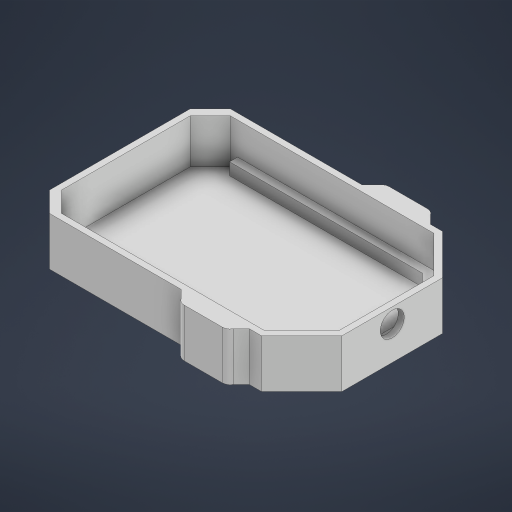
# Autodesk Inventor part: RC5 Controller
Saved by Autodesk Inventor 2024 (Build 280153000, 153)
## iProperties
Created: 2024-03-14
Part Number: RC5 Controller
Material: Generic
Document SubType Name: Modeling
Designer: MenMe
Density: 1 g/cm^3
Appearance: Default
Author: MenMe
Autodesk Inventor part; units mm, degrees
ref_plane "YZ Plane" through (0, 0, 0) normal (1, 0, 0) x (0, 1, 0)
ref_plane "XZ Plane" through (0, 0, 0) normal (0, 1, 0) x (-1, 0, 0)
ref_plane "XY Plane" through (0, 0, 0) normal (0, 0, 1) x (1, 0, 0)
sketch "Sketch1" plane through (0, 0, 0) normal (0, 1, 0) x (-1, 0, 0)
  line L0 (67.75, 0) -> (67.75, -45)
  line L1 (67.75, -45) -> (10, -45)
  line L2 (10, -45) -> (0, -35)
  line L3 (0, -35) -> (0, -10)
  line L4 (0, -10) -> (10, 0)
  line L5 (67.75, 0) -> (10, 0)
  line L6 (28, 0) -> (28, 3)
  line L7 (28, 3) -> (15, 3)
  line L8 (15, 3) -> (15, 0)
  line L9 (28, -45) -> (28, -48)
  line L10 (28, -48) -> (15, -48)
  line L11 (15, -48) -> (15, -45)
  line L12 (58, -48) -> (45, -48)
  line L13 (58, -45) -> (58, -48)
  line L14 (45, -48) -> (45, -45)
  line L15 (58, 0) -> (58, 3)
  line L16 (58, 3) -> (45, 3)
  line L17 (45, 3) -> (45, 0)
  point P0 (0, 0)
  point P1 (21.5, -48)
  point P2 (51.5, -48)
  dimension "d0" = 45
  dimension "d4" = 45
  dimension "d5" = 45
  dimension "d6" = 25
  dimension "d24" = 5
  dimension "d25" = 13
  dimension "d26" = 3
  dimension "d34" = 3
  dimension "d83" = 5
  dimension "d145" = 67.75
  dimension "d148" = 30
  dimension "d155" = 30
  constraints: 36 end point, 8 perpendicular, 6 point on line, 2 equal length, 2 horizontal, 1 midpoint, 16 other
  measures "d0" distance of L0.start L0.end
  measures "d4" angle of L2 L3
  measures "d5" angle of L4 L3
  measures "d6" distance of L2.end L3.end
  measures "d24" distance from line of L1.end L11
  measures "d25" distance of L9.end L10.end
  measures "d26" distance from line of L1 point (21.5, -48)
  measures "d34" distance between parallel lines of L5 L7
  measures "d83" distance from line of L4.end L8
  measures "d145" distance between parallel lines of L0 L3
  measures "d148" distance of L9.end L12.start
  measures "d155" distance of L6.start L15.start
extrude "Extrusion1" add sketch "Sketch1" along normal blind 12 contours L0 L1 L2 L3 L4 L5 | L5 L8 L7 L6 | L9 L10 L11 L1
sketch "Sketch2" plane through (0, 12, 0) normal (0, 1, 0) x (1, 0, 0)
  line L0 (-67.75, 0) -> (-28, 0) projected
  line L1 (-28, 0) -> (-28, -3) projected
  line L2 (-28, -3) -> (-15, -3) projected
  line L3 (-15, -3) -> (-15, 0) projected
  line L4 (-15, 0) -> (-10, 0) projected
  line L5 (-10, 0) -> (0, 10) projected
  line L6 (0, 10) -> (0, 35) projected
  line L7 (0, 35) -> (-10, 45) projected
  line L8 (-10, 45) -> (-15, 45) projected
  line L9 (-15, 45) -> (-15, 48) projected
  line L10 (-15, 48) -> (-28, 48) projected
  line L11 (-28, 48) -> (-28, 45) projected
  line L12 (-28, 45) -> (-67.75, 45) projected
  line L13 (-67.75, 45) -> (-67.75, 0) projected
  line L14 (0, 35) -> (-10, 45) construction
  line L15 (-67.75, 0) -> (-28, 0) construction
  line L16 (-66.25, 43.5) -> (-66.25, 1.5)
  line L17 (-66.25, 1.5) -> (-10.6213, 1.5)
  line L18 (-10.6213, 1.5) -> (-1.5, 10.6213)
  line L19 (-1.5, 10.6213) -> (-1.5, 34.3787)
  line L20 (-1.5, 34.3787) -> (-10.6213, 43.5)
  line L21 (-10.6213, 43.5) -> (-66.25, 43.5)
  line L22 (-10, 0) -> (0, 10) construction
  point P0 (0, 0)
  point P1 (-40, 0)
  point P2 (-66.25, 22.5)
  point P3 (-67.75, 22.5)
  dimension "d126" = 42
  dimension "d132" = 1.5
  dimension "d133" = 1.5
  dimension "d134" = 1.5
  constraints: 12 end point, 4 parallel, 3 perpendicular, 2 midpoint, 1 horizontal alignment, 1 vertical
  measures "d126" distance between parallel lines of L21 L17
  measures "d132" distance between parallel lines of L13 L16
  measures "d133" distance between parallel lines of L6 L19
  measures "d134" distance between parallel lines of L7 L20
extrude "Extrusion2" cut sketch "Sketch2" against normal blind 11 contours L21 L20 L19 L18 L17 L16
chamfer "Chamfer1" distance 2 angle 45 4 edges at (-28, 6, 0) (-15, 6, 0) (-15, 6, -45) (-28, 6, -45)
chamfer "Chamfer2" distance 5 angle 45 4 edges at (-67.75, 6, -45) (-66.25, 6.5, -43.5) (-67.75, 6, 0) (-66.25, 6.5, -1.5)
sketch "Sketch3" plane through (0, 0, -10) normal (1, 0, 0) x (0, 0, -1)
  line L0 (0, 0) -> (0, 12) projected
  line L1 (25, 0) -> (25, 12) projected
  line L2 (0, 0) -> (25, 0) projected
  circle A0 centre (12.5, 8.3) radius 3
  point P0 (-10, 0)
  dimension "d93" = 6
  dimension "d94" = 12.5
  dimension "d95" = 8.3
  constraints: 1 centre point
  measures "d93" diameter of A0
  measures "d94" distance from line of L1 A0.centre
  measures "d95" distance from line of L2 A0.centre
extrude "Extrusion3" cut sketch "Sketch3" against normal blind 8
fillet "Fillet1" radius 2 4 edges at (-28, 6, -48) (-15, 6, -48) (-15, 6, 3) (-28, 6, 3)
sketch "Sketch5" plane through (0, 1, 0) normal (0, 1, 0) x (1, 0, 0)
  line L0 (-103.5, 43.5) -> (-10.6213, 43.5) projected
  line L1 (-10.6213, 1.5) -> (-103.5, 1.5) projected
  line L2 (-108.5, 6.5) -> (-103.5, 1.5) projected
  line L3 (-10.6213, 1.5) -> (-103.5, 1.5) projected
  line L4 (-1.5, 10.6213) -> (-10.6213, 1.5) projected
  line L5 (-1.5, 34.3787) -> (-1.5, 10.6213) projected
  line L6 (-10.6213, 43.5) -> (-1.5, 34.3787) projected
  line L7 (-103.5, 43.5) -> (-10.6213, 43.5) projected
  line L8 (-103.5, 43.5) -> (-108.5, 38.5) projected
  line L9 (-108.5, 6.5) -> (-108.5, 38.5) projected
  line L10 (-10.6213, 1.5) -> (-1.5, 10.6213)
  line L11 (-1.5, 34.3787) -> (-1.5, 10.6213)
  line L12 (-1.5, 34.3787) -> (-10.6213, 43.5)
  line L13 (-10.6213, 43.5) -> (-59.4466, 43.5)
  line L14 (-59.4466, 43.5) -> (-59.4466, 1.5)
  line L15 (-59.4466, 1.5) -> (-10.6213, 1.5)
  line L16 (-3.5, 11.4497) -> (-11.4497, 3.5)
  line L17 (-11.4497, 3.5) -> (-102.6716, 3.5)
  line L18 (-102.6716, 3.5) -> (-106.5, 7.3284)
  line L19 (-106.5, 7.3284) -> (-106.5, 37.6716)
  line L20 (-106.5, 37.6716) -> (-102.6716, 41.5)
  line L21 (-102.6716, 41.5) -> (-11.4497, 41.5)
  line L22 (-11.4497, 41.5) -> (-3.5, 33.5503)
  line L23 (-3.5, 33.5503) -> (-3.5, 11.4497)
  point P0 (0, 0)
  point P1 (-59.4466, 1.5)
  point P2 (-10.6213, 43.5)
  point P3 (-59.4466, 3.5)
  point P4 (-59.4466, 41.5)
  dimension "d109" = 2
  constraints: 28 end point, 3 perpendicular, 2 collinear, 2 point on line, 7 other
  measures "d109" distance between parallel lines of L5 L23
extrude "Extrusion4" add sketch "Sketch5" along normal blind 3 contours L0 L6 L5 L4 L1 L14 L17 L16 L23 L22 L21
body "Solid1"
